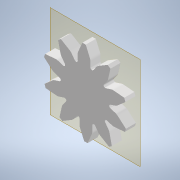
# Autodesk Inventor part: Pinion
Saved by Autodesk Inventor 2020 (Build 240168000, 168)
## iProperties
Created: 2020-12-28
Part Number: Pinion
Material: Generic
Document SubType Name: Modeling
Designer: moham
Density: 1 g/cm^3
Appearance: Default
Author: moham
Autodesk Inventor part; units mm, degrees
ref_plane "YZ Plane" through (0, 0, 0) normal (1, 0, 0) x (0, 1, 0)
ref_plane "XZ Plane" through (0, 0, 0) normal (0, 1, 0) x (-1, 0, 0)
ref_plane "XY Plane" through (0, 0, 0) normal (0, 0, 1) x (1, 0, 0)
sketch "Sketch2" plane through (0, 0, 0) normal (0, 0, 1) x (1, 0, 0)
  point P0 (0, 0)
sketch "Sketch3" plane through (0, 0, 0) normal (0, 0, 1) x (1, 0, 0)
  line L0 (3, 23.7889) -> (-2.507, 23.7889)
  circle A0 centre (0, 0) radius 19
  circle A1 centre (0, 0) radius 18
  arc A2 (-1, 19) -> (1, 19) centre (0, 19) ccw
  line L1 (-2.507, 23.7889) -> (-3, 23.7889)
  arc A3 (-0.9997, 18.9737) -> (-3, 23.7889) centre (-7.9849, 18.8949) ccw
  arc A4 (3, 23.7889) -> (0.9997, 18.9737) centre (7.9849, 18.8949) ccw
  dimension "d12" = 5.507
  constraints: 13 point on circle, 5 centre point, 4 end point, 1 coincident, 1 horizontal
  measures "d12" distance of L0.start L0.end
sketch "Sketch4" plane through (0, 0, 0) normal (0, 0, 1) x (1, 0, 0)
  line L0 (-12, 23.7889) -> (198, 23.7889)
  line L1 (198, 23.7889) -> (198, 16.7889)
  line L2 (198, 16.7889) -> (-12, 16.7889)
  line L3 (-12, 16.7889) -> (-12, 23.7889)
  point P0 (0, 0)
  point P1 (-3, 23.7889)
  point P2 (3, 23.7889)
  dimension "d13" = 210
  dimension "d14" = 7
  dimension "d15" = 9
  constraints: 8 end point, 2 parallel, 1 horizontal, 1 perpendicular, 1 point on line
  measures "d13" distance of L1.end L2.end
  measures "d14" distance of L0.end L1.end
  measures "d15" distance from line of point (-3, 23.789) L3
extrude "Extrusion2" add sketch "Sketch4" against normal blind 6
extrude "Extrusion3" cut sketch "Sketch3" against normal blind 6 contours A4 A2 A0 A3 L1 L0
pattern_linear "Rectangular Pattern1" count 31 spacing 6.2 along (1, 0, 0) of "Extrusion3"
sketch "Sketch5" plane through (198, 16.7889, 0) normal (1, 0, 0) x (0, 0, -1)
  line L0 (0, 0) -> (6, 0) projected
  point P0 (3, 0)
  constraints: 2 end point, 1 midpoint
body "Solid2"
